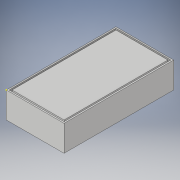
# Autodesk Inventor part: rev1 base
Saved by Autodesk Inventor 2017 (Build 210142000, 142)
## iProperties
Created: 2019-05-03
Part Number: rev1 base
Material: Generic
Document SubType Name: Modeling
Designer: Roman
Density: 1 g/cm^3
Appearance: Default
Author: Roman
Autodesk Inventor part; units mm, degrees
ref_plane "YZ Plane" through (0, 0, 0) normal (1, 0, 0) x (0, 1, 0)
ref_plane "XZ Plane" through (0, 0, 0) normal (0, 1, 0) x (-1, 0, 0)
ref_plane "XY Plane" through (0, 0, 0) normal (0, 0, 1) x (1, 0, 0)
sketch "Sketch1" plane through (0, 0, 0) normal (0, 1, 0) x (-1, 0, 0)
  line L0 (0, 0) -> (-1016, 0)
  line L1 (-1016, 0) -> (-1016, -1930.4)
  line L2 (-1016, -1930.4) -> (0, -1930.4)
  line L3 (0, -1930.4) -> (0, 0)
  dimension "d0" = 1016
  dimension "d1" = 1930.4
  constraints: 8 end point, 2 parallel, 1 horizontal, 1 perpendicular
  measures "d0" distance of L2.end L1.end
  measures "d1" distance of L1.end L0.end
extrude "Extrusion1" add sketch "Sketch1" along normal blind 457.2
sketch "Sketch8" plane through (0, 457.2, 0) normal (0, 1, 0) x (1, 0, 0)
  line L0 (25.4, 25.4) -> (990.6, 25.4)
  line L1 (990.6, 25.4) -> (990.6, 1905)
  line L2 (990.6, 1905) -> (25.4, 1905)
  line L3 (25.4, 1905) -> (25.4, 25.4)
  line L4 (50.8, 50.8) -> (965.2, 50.8)
  line L5 (965.2, 50.8) -> (965.2, 1879.6)
  line L6 (965.2, 1879.6) -> (50.8, 1879.6)
  line L7 (50.8, 1879.6) -> (50.8, 50.8)
  line L8 (50.8, 965.2) -> (25.4, 965.2)
  line L9 (965.2, 965.2) -> (990.6, 965.2)
  line L10 (508, 1879.6) -> (508, 1905)
  line L11 (508, 50.8) -> (508, 25.4)
  line L12 (508, 25.4) -> (508, 0)
  line L13 (0, 0) -> (1016, 0) projected
  line L14 (508, 1905) -> (508, 1930.4)
  line L15 (1016, 1930.4) -> (0, 1930.4) projected
  line L16 (25.4, 965.2) -> (0, 965.2)
  line L17 (0, 1930.4) -> (0, 0) projected
  line L18 (990.6, 965.2) -> (1016, 965.2)
  line L19 (1016, 0) -> (1016, 1930.4) projected
  dimension "d13" = 25.4
  dimension "d14" = 25.4
  dimension "d15" = 25.4
  dimension "d16" = 25.4
  constraints: 32 end point, 12 midpoint, 4 collinear, 4 parallel, 2 horizontal, 2 perpendicular, 1 vertical
  measures "d13" distance of L11.start L11.end
  measures "d14" distance of L9.start L9.end
  measures "d15" distance of L9.end L18.end
  measures "d16" distance of L11.end L12.end
extrude "Extrusion3" cut sketch "Sketch8" against normal blind 50.8 contours L3 L8 L7 L4 L11 L0 | L11 L4 L5 L9 L1 L0 | L3 L2 L10 L6 L7 L8 | L9 L5 L6 L10 L2 L1
sketch "InnerInset1" plane through (0, 406.4, 0) normal (0, 1, 0) x (1, 0, 0)
  line L0 (25.4, 25.4) -> (25.4, 1905) projected
  line L1 (50.8, 1879.6) -> (50.8, 50.8) projected
  line L2 (25.4, 279.4) -> (50.8, 279.4)
  line L3 (50.8, 279.4) -> (50.8, 736.6)
  line L4 (50.8, 736.6) -> (25.4, 736.6)
  line L5 (25.4, 736.6) -> (25.4, 279.4)
  line L6 (990.6, 25.4) -> (25.4, 25.4) projected
  line L7 (25.4, 1193.8) -> (50.8, 1193.8)
  line L8 (50.8, 1193.8) -> (50.8, 1651)
  line L9 (50.8, 1651) -> (25.4, 1651)
  line L10 (25.4, 1651) -> (25.4, 1193.8)
  line L11 (25.4, 1905) -> (990.6, 1905) projected
  point P0 (0, 0)
  dimension "d19" = 254
  dimension "d20" = 457.2
  dimension "d21" = 457.2
  dimension "d22" = 254
  constraints: 16 end point, 4 parallel, 4 point on line, 2 horizontal, 2 perpendicular
  measures "d19" distance between parallel lines of L6 L2
  measures "d20" distance between parallel lines of L2 L4
  measures "d21" distance between parallel lines of L9 L7
  measures "d22" distance between parallel lines of L11 L9
extrude "Extrusion4" cut sketch "InnerInset1" against normal blind 50.8 contours L0 L4 L1 L2 | L0 L9 L1 L7
ref_plane "Work Plane1" through (508, 0, 0) normal (1, 0, 0) x (0, 0, -1)
mirror "Mirror1" about plane through (508, 0, 0) normal (1, 0, 0) of "Extrusion4"
ref_plane "Work Plane2" through (1016, 0, -965.2) normal (0, 0, -1) x (-1, 0, 0)
sketch "Sketch10" plane through (0, 406.4, 0) normal (0, 1, 0) x (1, 0, 0)
  line L0 (50.8, 50.8) -> (965.2, 50.8) projected
  line L1 (990.6, 25.4) -> (25.4, 25.4) projected
  line L2 (203.2, 50.8) -> (355.6, 50.8)
  line L3 (355.6, 50.8) -> (355.6, 25.4)
  line L4 (355.6, 25.4) -> (203.2, 25.4)
  line L5 (203.2, 25.4) -> (203.2, 50.8)
  line L6 (660.4, 50.8) -> (812.8, 50.8)
  line L7 (812.8, 50.8) -> (812.8, 25.4)
  line L8 (812.8, 25.4) -> (660.4, 25.4)
  line L9 (660.4, 25.4) -> (660.4, 50.8)
  line L10 (203.2, 38.1) -> (355.6, 38.1)
  line L11 (660.4, 38.1) -> (812.8, 38.1)
  line L12 (25.4, 25.4) -> (25.4, 1905) projected
  line L13 (990.6, 1905) -> (990.6, 25.4) projected
  point P0 (0, 0)
  dimension "d25" = 177.8
  dimension "d26" = 177.8
  dimension "d27" = 152.4
  constraints: 20 end point, 4 midpoint, 4 parallel, 4 point on line, 2 horizontal, 2 perpendicular, 1 collinear
  measures "d25" distance from line of L12 L10.start
  measures "d26" distance from line of L13 L11.end
  measures "d27" distance of L11.start L11.end
extrude "Extrusion5" cut sketch "Sketch10" against normal blind 50.8 contours L0 L3 L10 L5 | L10 L3 L1 L5 | L0 L7 L11 L9 | L11 L7 L1 L9
mirror "Mirror2" about plane through (1016, 0, -965.2) normal (0, 0, -1) of "Extrusion5"
sketch "Sketch11" plane through (0, 457.2, 0) normal (0, 1, 0) x (1, 0, 0)
  point P0 (0, 0)
body "Solid1"
